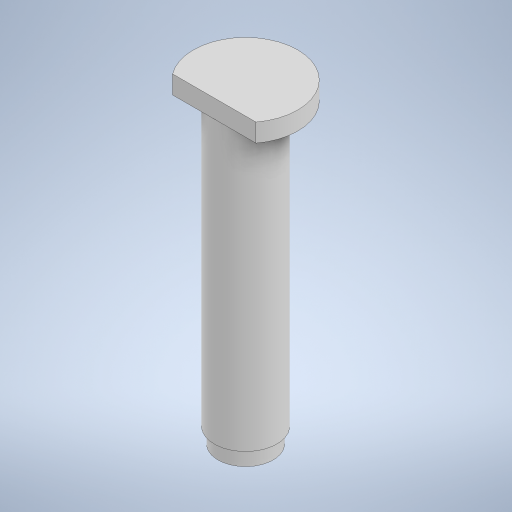
# Autodesk Inventor part: shim_peg_V3
Saved by Autodesk Inventor 2024.3 (Build 283343000, 343)
## iProperties
Created: 2024-04-09
Part Number: shim_peg_V3
Material: Generic
Document SubType Name: Modeling
Designer: Joshua Harper
Density: 1 g/cm^3
Appearance: Default
Author: Joshua Harper
Autodesk Inventor part; units mm, degrees
ref_plane "YZ Plane" through (0, 0, 0) normal (1, 0, 0) x (0, 1, 0)
ref_plane "XZ Plane" through (0, 0, 0) normal (0, 1, 0) x (-1, 0, 0)
ref_plane "XY Plane" through (0, 0, 0) normal (0, 0, 1) x (1, 0, 0)
sketch "Sketch1" plane through (0, 0, 0) normal (0, 0, 1) x (1, 0, 0)
  line L0 (0, 0) -> (0, 39.4806) construction
  line L1 (0, 0) -> (-3, 0) construction
  line L2 (-3, 0) -> (-3, 27)
  line L3 (-3, 27) -> (-5, 27)
  line L4 (-5, 27) -> (-5, 28.75)
  line L5 (0, 0) -> (0, 29)
  line L6 (-3, 0) -> (-2.65, 0)
  line L7 (-2.65, -1.5) -> (0, -1.5)
  line L8 (0, -1.5) -> (0, 0)
  line L9 (-2.65, 0) -> (-2.65, -1.5)
  line L10 (-5, 28.75) -> (0, 28.75)
  dimension "d0" = 3
  dimension "d1" = 5
  dimension "d5" = 27
  dimension "d12" = 2.65
  dimension "d13" = 1.5
  dimension "d24" = 1.75
  constraints: 23 end point, 4 perpendicular, 3 horizontal, 3 point on line, 2 vertical
  measures "d0" distance between parallel lines of L0 L2
  measures "d1" distance between parallel lines of L0 L4
  measures "d5" distance from line of L1.end L3
  measures "d12" distance between parallel lines of L8 L9
  measures "d13" distance between parallel lines of L7 L1
  measures "d24" distance between parallel lines of L10 L3
revolve "Revolution1" add sketch "Sketch1" angle 360 about axis through (0, 0, 0) along (0, 1, 0)
sketch "Sketch3" plane through (0, -1.5, 0) normal (0, -1, 0) x (1, 0, 0)
  point P0 (0, 0)
  point P1 (0, 0)
  constraints: 1 coincident
hole "Hole1" at (0, -1.5, 0) direction (0, 1, 0) diameter 3.242 depth 11.8 tip angle 118 thread size "M4x0.7" class "6H" standard "ANSI Metric M Profile"
sketch "Sketch4" plane through (0, 27, 0) normal (0, -1, 0) x (1, 0, 0)
  arc A0 (4, 3) -> (-4, 3) centre (0, 0) ccw
  line L0 (-4, 3) -> (4, 3)
  circle A1 centre (0, 0) radius 3 projected
  circle A2 centre (0, 0) radius 5 projected
  constraints: 2 end point, 2 point on circle, 1 centre point, 1 coincident, 1 concentric, 1 horizontal, 1 tangent
extrude "Extrusion2" cut sketch "Sketch4" against normal through all contours L0 A0
body "Solid1"
